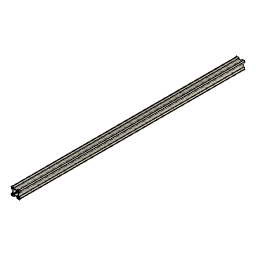
assemblage+liaison+fonctionnelle (Autodesk Fusion 360 archive; units mm, degrees)
design "profil 24*24*623mm"
Autodesk Fusion 360 part; units mm, degrees
sketch "Esquisse1" plane through (0, 0, 0) normal (0, 1, 0) x (1, 0, 0)
  line L0 (12, 12) -> (-12, 12) construction
  line L1 (-12, 12) -> (-12, -12) construction
  line L2 (-12, -12) -> (12, -12) construction
  line L3 (12, -12) -> (12, 12) construction
  line L4 (12, 12) -> (-12, -12) construction
  line L5 (-12, 12) -> (12, -12) construction
  line L6 (6, -6) -> (-6, -6)
  line L7 (-6, -6) -> (-6, 6)
  line L8 (-6, 6) -> (6, 6)
  line L9 (6, 6) -> (6, -6)
  line L10 (6, -6) -> (-6, 6) construction
  line L11 (-6, -6) -> (6, 6) construction
  line L12 (8, -8) -> (-8, -8)
  line L13 (-8, -8) -> (-8, 8)
  line L14 (-8, 8) -> (8, 8)
  line L15 (8, 8) -> (8, -8)
  line L16 (8, -8) -> (-8, 8) construction
  line L17 (-8, -8) -> (8, 8) construction
  circle A0 centre (0, 0) radius 7.2111
  circle A1 centre (-8.818, -8.818) radius 1.5
  circle A2 centre (-10.25, -10.25) radius 1.75
  circle A3 centre (-7.0251, -9.5) radius 2.5
  line L18 (-9.0126, -11.4874) -> (-8.7929, -11.2678)
  line L19 (-8.7929, -11.2678) -> (-8.0607, -12) construction
  line L20 (-4.5251, -9.5) -> (-4.5251, -8) construction
  line L21 (-4.5251, -9.5) -> (-6.25, -9.5)
  line L22 (-6.25, -9.5) -> (-6.25, -8)
  circle A4 centre (-9.5, -7.0251) radius 2.5
  line L23 (-11.4874, -9.0126) -> (-11.2678, -8.7929)
  line L24 (-9.5, -4.5251) -> (-9.5, -6.25)
  line L25 (-9.5, -6.25) -> (-8, -6.25)
  circle A5 centre (10.25, -10.25) radius 1.75
  circle A6 centre (7.0251, -9.5) radius 2.5
  circle A7 centre (8.818, -8.818) radius 1.5
  circle A8 centre (9.5, -7.0251) radius 2.5
  line L26 (9.5, -4.5251) -> (9.5, -6.25)
  line L27 (9.5, -6.25) -> (8, -6.25)
  line L28 (6.25, -9.5) -> (6.25, -8)
  line L29 (4.5251, -9.5) -> (6.25, -9.5)
  line L30 (9.0126, -11.4874) -> (8.7929, -11.2678)
  line L31 (11.4874, -9.0126) -> (11.2678, -8.7929)
  circle A9 centre (10.25, 10.25) radius 1.75
  circle A10 centre (9.5, 7.0251) radius 2.5
  circle A11 centre (8.818, 8.818) radius 1.5
  circle A12 centre (7.0251, 9.5) radius 2.5
  line L32 (4.5251, 9.5) -> (6.25, 9.5)
  line L33 (6.25, 9.5) -> (6.25, 8)
  line L34 (9.5, 6.25) -> (8, 6.25)
  line L35 (9.5, 4.5251) -> (9.5, 6.25)
  line L36 (11.4874, 9.0126) -> (11.2678, 8.7929)
  line L37 (9.0126, 11.4874) -> (8.7929, 11.2678)
  circle A13 centre (-10.25, 10.25) radius 1.75
  circle A14 centre (-7.0251, 9.5) radius 2.5
  circle A15 centre (-8.818, 8.818) radius 1.5
  circle A16 centre (-9.5, 7.0251) radius 2.5
  line L38 (-9.5, 4.5251) -> (-9.5, 6.25)
  line L39 (-9.5, 6.25) -> (-8, 6.25)
  line L40 (-6.25, 9.5) -> (-6.25, 8)
  line L41 (-4.5251, 9.5) -> (-6.25, 9.5)
  line L42 (-9.0126, 11.4874) -> (-8.7929, 11.2678)
  line L43 (-11.4874, 9.0126) -> (-11.2678, 8.7929)
  point P0 (-4, -6)
  point P1 (-8.7929, -11.2678)
  dimension "d1" = 24
  dimension "d2" = 24
  dimension "d3" = 2
  dimension "d5" = 2
  dimension "d12" = 3
  dimension "d19" = 3.5
  dimension "d20" = 5
  dimension "d22" = 360
  dimension "d25" = 4.5
  dimension "d26" = 1.5
  dimension "d27" = 12.5
  constraint horizontal L0
  constraint perpendicular L0 L1
  constraint parallel L0 L2
  constraint parallel L1 L3
  constraint coincident L4 A0.centre
  constraint coincident L5 A0.centre
  constraint coincident A0.centre origin
  constraint horizontal L6
  constraint perpendicular L6 L7
  constraint parallel L6 L8
  constraint parallel L7 L9
  constraint coincident L10 A0.centre
  constraint coincident L11 A0.centre
  constraint coincident L5 L6.start
  constraint horizontal L12
  constraint perpendicular L12 L13
  constraint parallel L12 L14
  constraint parallel L13 L15
  constraint coincident L16 A0.centre
  constraint coincident L17 A0.centre
  constraint coincident L5 L12.start
  constraint coincident A0 P0
  constraint coincident L6 P0
  constraint coincident L4 A1.centre
  constraint coincident L4 A2.centre
  constraint tangent L2 A2
  constraint tangent L2 A3
  constraint coincident A2 L18.start
  constraint tangent A2 L18
  constraint parallel L4 L18
  constraint coincident L18 P1
  constraint perpendicular L18 L19
  constraint tangent A3 L19
  constraint coincident P1 L18.end
  constraint coincident L2 L19.end
  constraint coincident A3 P1
  constraint coincident A3 L20.start
  constraint coincident L12 L20.end
  constraint tangent A3 L20
  constraint perpendicular L12 L20
  constraint perpendicular L20 L21
  constraint coincident L12 L22.end
  constraint perpendicular L12 L22
  constraint symmetric L4 A3 A4
  constraint symmetric L4 L18.start L23.start
  constraint symmetric L4 P1 L23.end
  constraint symmetric L4 L20.start L24.start
  constraint symmetric L4 L21.end L24.end
  constraint symmetric L4 L22.end L25.end
  measures "d1" distance of L1.end L2.end
  measures "d2" distance of L0.end L1.end
  measures "d3" distance of L7 L13
  measures "d5" distance of L6.end P0
  measures "d12" diameter of A1
  measures "d19" diameter of A2
  measures "d20" diameter of A3
  measures "d25" distance of L1.end A1.centre
  measures "d26" distance of L21.end L22.end
  measures "d27" distance of L22 L28
extrude "Extrusion1" add sketch "Esquisse1" along normal blind 623 contours L12 A7 A8 | L12 L15 A6 A7 A8 | L15 A6 A7 | L12 A5 A6 A7 A8 L28 L29 | L12 A6 A8 | L15 A6 A8 | L15 A5 A6 A7 A8 L26 L27 | L12 L13 L14 L15 A3 A4 A6 A8 A10 A12 A14 A16 | A5 A6 A7 | A5 A7 A8 | A5 A6 A7 A8 | A5 A6 L30 | A5 A8 L31 | L12 A3 A4 | L15 A10 A12 | L12 A1 A2 A3 L21 L22 A4 | L12 L13 A1 A3 A4 | L13 A3 A4 | L15 A9 A10 A11 A12 L34 L35 | L14 A10 A12 | L14 L15 A10 A11 A12 | L12 A1 A4 | A2 A3 L18 | L13 A1 A2 A3 A4 L24 L25 | L13 A1 A3 | L15 A11 A12 | L14 A10 A11 | L14 A9 A10 A11 A12 L32 L33 | A1 A2 A3 | A1 A2 A3 A4 | L13 A14 A16 | L14 A14 A16 | A9 A10 L36 | A2 A4 L23 | A1 A2 A4 | L13 A13 A14 A15 A16 L38 L39 | L13 L14 A14 A15 A16 | A9 A10 A11 | A9 A11 A12 | L14 A13 A14 A15 A16 L40 L41 | A9 A12 L37 | A9 A10 A11 A12 | L13 A14 A15 | A13 A16 L43 | L14 A15 A16 | A13 A14 L42 | A13 A15 A16 | A13 A14 A15 A16 | A13 A14 A15 picked at (8.883, -10.6208) picked at (10.6212, -8.8632) picked at (10.8484, -9.818) picked at (-8.883, -10.6208) picked at (-10.851, -9.7977) picked at (-10.6208, -8.883) picked at (10.6212, 8.8632) picked at (8.883, 10.6208) picked at (10.8484, 9.818) picked at (-10.6208, 8.883) picked at (-9.7977, 10.851) picked at (-8.883, 10.6208)
